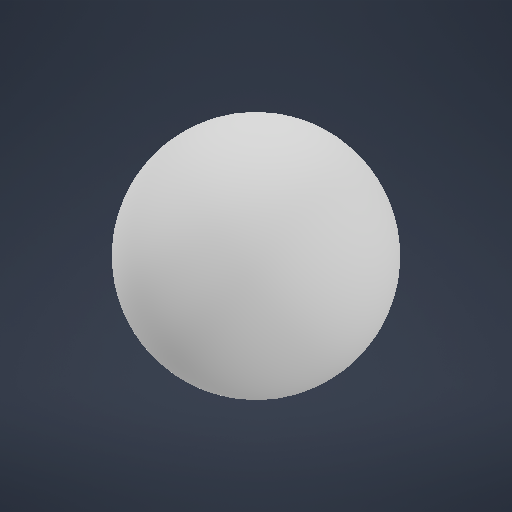
# Autodesk Inventor part: BumperCaster
Saved by Autodesk Inventor 2026.1 (Build 301233000, 233)
## iProperties
Created: 2026-06-30
Part Number: BumperCaster
Material: Generic
Document SubType Name: Modeling
Designer: Kasi Pusuluri
Density: 1 g/cm^3
Appearance: Default
Author: Kasi Pusuluri
Autodesk Inventor part; units mm, degrees
ref_plane "YZ Plane" through (0, 0, 0) normal (1, 0, 0) x (0, 1, 0)
ref_plane "XZ Plane" through (0, 0, 0) normal (0, 1, 0) x (-1, 0, 0)
ref_plane "XY Plane" through (0, 0, 0) normal (0, 0, 1) x (1, 0, 0)
sketch "Sketch1" plane through (0, 0, 0) normal (0, 1, 0) x (-1, 0, 0)
  line L0 (12.7529, 0) -> (-10.4019, 0)
  arc A0 (-8.89, 0) -> (8.89, 0) centre (0, 0) ccw
  dimension "d1" = 90
  constraints: 2 end point, 2 point on circle, 2 point on line, 1 centre point, 1 horizontal
revolve "Revolution1" add sketch "Sketch1" angle 360 about axis through (-12.7529, 0, 0) along (1, 0, 0)
body "Solid1"
